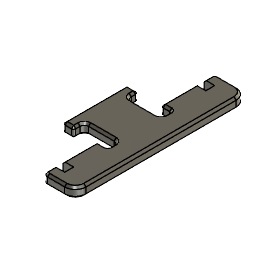
Rubber Band Holder (Autodesk Fusion 360 design; units mm, degrees)
Autodesk Fusion 360 part; units mm, degrees
sketch "Sketch1" plane through (0, 0, 0) normal (0, 0, 1) x (1, 0, 0)
  line L0 (7.5, -40.2) -> (-7.5, -40.2)
  line L1 (-7.5, -40.2) -> (-7.5, 40.2)
  line L2 (-7.5, 40.2) -> (7.5, 40.2)
  line L3 (7.5, 40.2) -> (7.5, -40.2)
  line L4 (7.5, -40.2) -> (-7.5, 40.2) construction
  line L5 (-7.5, -40.2) -> (7.5, 40.2) construction
  line L6 (-7.5, 35.2) -> (-2.5, 35.2)
  line L7 (-2.5, 35.2) -> (-2.5, 31)
  line L8 (-2.5, 31) -> (-7.5, 31)
  line L9 (-7.5, 31) -> (-7.5, 35.2)
  line L10 (-7.5, -31) -> (-2.5, -31)
  line L11 (-2.5, -31) -> (-2.5, -35.2)
  line L12 (-2.5, -35.2) -> (-7.5, -35.2)
  line L13 (-7.5, -35.2) -> (-7.5, -31)
  line L14 (-2.5, 10) -> (-18.5, 10)
  line L15 (-18.5, 10) -> (-18.5, -10)
  line L16 (-18.5, -10) -> (-2.5, -10)
  line L17 (-2.5, -10) -> (-2.5, 10)
  line L18 (-23.5, 15) -> (-18.5, 15)
  line L19 (-18.5, 15) -> (-18.5, -15)
  line L20 (-18.5, -15) -> (-23.5, -15)
  line L21 (-23.5, -15) -> (-23.5, 15)
  line L22 (-2.5, -10) -> (-2.5, -15)
  line L23 (-2.5, -15) -> (-7.5, -15)
  line L24 (-2.5, 10) -> (-2.5, 15)
  line L25 (-2.5, 15) -> (-7.5, 15)
  dimension "d1" = 80.4
  dimension "d2" = 15
  dimension "d3" = 5
  dimension "d4" = 4.2
  dimension "d5" = 5
  dimension "d6" = 4.2
  dimension "d7" = 5
  dimension "d8" = 5
  dimension "d9" = 16
  dimension "d10" = 5
  dimension "d11" = 5
  dimension "d12" = 5
  dimension "d13" = 30
  dimension "d14" = 5
  dimension "d15" = 20
  dimension "d16" = 10
  dimension "d26" = 5
  dimension "d27" = 5
  constraint horizontal L0
  constraint perpendicular L0 L1
  constraint parallel L0 L2
  constraint parallel L1 L3
  constraint coincident L4 origin
  constraint coincident L5 origin
  constraint horizontal L6
  constraint vertical L7
  constraint horizontal L8
  constraint vertical L9
  constraint coincident L1 L6.start
  constraint horizontal L10
  constraint vertical L11
  constraint horizontal L12
  constraint vertical L13
  constraint coincident L1 L10.start
  constraint horizontal L14
  constraint vertical L15
  constraint horizontal L16
  constraint vertical L17
  constraint horizontal L18
  constraint vertical L19
  constraint horizontal L20
  constraint vertical L21
  constraint perpendicular L16 L22
  constraint coincident L1 L23.end
  constraint perpendicular L1 L23
  constraint perpendicular L14 L24
  constraint coincident L1 L25.end
  constraint perpendicular L1 L25
  measures "d1" distance of L0.end L1.end
  measures "d2" distance of L0.start L0.end
  measures "d3" distance of L6.start L6.end
  measures "d4" distance of L6.start L8.end
  measures "d5" distance of L10.start L10.end
  measures "d6" distance of L10.start L12.end
  measures "d7" distance of L0 L12
  measures "d8" distance of L2 L6
  measures "d9" distance of L15.end L16.end
  measures "d10" distance of L1 L17
  measures "d11" distance of L18.start L18.end
  measures "d12" distance of L15 L21
  measures "d13" distance of L18.start L20.end
  measures "d14" distance of L14 L18
  measures "d15" distance of L14.start L16.end
  measures "d16" distance of origin L14
  measures "d26" distance of L14.start L24.end
  measures "d27" distance of L16.end L22.end
extrude "Extrude1" add sketch "Sketch1" along normal blind 4.8 contours L0 L1 L2 L3 L6 L7 L8 L10 L11 L12 L17 L22 L23 L24 L25 | L1 L14 L15 L16 L19 | L1 L14 L16 L17 | L15 L18 L19 L20 L21
fillet "Fillet1" radius 5 2 edges at (7.5, 40.2, 2.4) (7.5, -40.2, 2.4)
fillet "Fillet1" radius 2 6 edges at (-18.5, 10, 2.4) (-18.5, -10, 2.4) (-7.5, 40.2, 2.4) (-7.5, -40.2, 2.4) (-2.5, -10, 2.4) (-2.5, 10, 2.4)
fillet "Fillet1" radius 1 8 edges at (-18.5, 15, 2.4) (-23.5, 15, 2.4) (-18.5, -15, 2.4) (-23.5, -15, 2.4) (-2.5, 15, 2.4) (-7.5, 15, 2.4) (-2.5, -15, 2.4) (-7.5, -15, 2.4)
chamfer "Chamfer1" distance 1 angle 45 28 edges at (-10.5, 10, 4.8) (-10.5, -10, 4.8) (-10.5, -10, 0) (-10.5, 10, 0) (7.5, 0, 4.8) (7.5, 0, 0) (-18.5, -12.5, 4.8) (-18.5, -12.5, 0) (-21, -15, 4.8) (-21, -15, 0) (-23.5, 0, 4.8) (-7.5, -23, 4.8) (-7.5, -23, 0) (-7.5, -37.7, 0) (0, -40.2, 0) (0, -40.2, 4.8) (0, 40.2, 4.8) (-7.5, 37.7, 4.8) (-7.5, 37.7, 0) (-7.5, 23, 4.8) (-7.5, 23, 0) (-7.5, -37.7, 4.8) (-23.5, 0, 0) (-21, 15, 0) (0, 40.2, 0) (-18.5, 12.5, 0) (-21, 15, 4.8) (-18.5, 12.5, 4.8)
equation "d12 = d11"
equation "d16 = d15 / 2"
equation "d26 = d14"
equation "d27 = d26"
